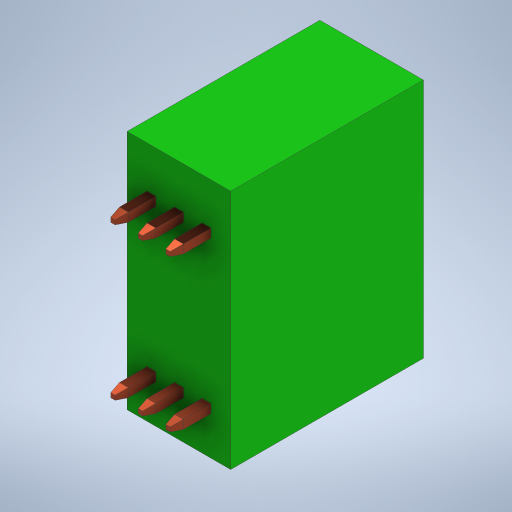
# Autodesk Inventor part: DB2EVH-2.5-2-3P-GN
Saved by Autodesk Inventor 2024 (Build 280153000, 153)
## iProperties
Created: 2023-05-23
Part Number: DB2EVH-2.5-2-3P-GN
Material: Generic
Document SubType Name: Modeling
Designer: torba
Density: 1 g/cm^3
Appearance: Default
Author: torba
Autodesk Inventor part; units mm, degrees
ref_plane "YZ Plane" through (0, 0, 0) normal (1, 0, 0) x (0, 1, 0)
ref_plane "XZ Plane" through (0, 0, 0) normal (0, 1, 0) x (-1, 0, 0)
ref_plane "XY Plane" through (0, 0, 0) normal (0, 0, 1) x (1, 0, 0)
sketch "Sketch1" plane through (0, 0, 0) normal (0, 0, 1) x (1, 0, 0)
  line L0 (0, 0) -> (9.4, 0)
  line L1 (9.4, 0) -> (9.4, -21.9)
  line L2 (9.4, -21.9) -> (0, -21.9)
  line L3 (0, -21.9) -> (0, 0)
  line L4 (1.8, -18.4) -> (2.6, -18.4)
  line L5 (2.6, -18.4) -> (2.6, -17.6)
  line L6 (2.6, -17.6) -> (1.8, -17.6)
  line L7 (1.8, -17.6) -> (1.8, -18.4)
  line L8 (1.8, -18.4) -> (2.6, -17.6) construction
  point P0 (2.2, -18)
  dimension "d0" = 9.4
  dimension "d1" = 21.9
  dimension "d2" = 0.8
  dimension "d3" = 0.8
  dimension "d5" = 3.9
  dimension "d6" = 2.2
  dimension "d14" = 0
  dimension "d15" = 0
  dimension "d22" = 7.2
  constraints: 18 end point, 4 parallel, 2 horizontal, 2 perpendicular, 1 midpoint
  measures "d0" distance between parallel lines of L1 L3
  measures "d1" distance between parallel lines of L2 L0
  measures "d2" distance of L4.end L5.end
  measures "d3" distance of L4.start L4.end
  measures "d5" distance from line of L2 point (2.2, -18)
  measures "d6" distance from line of L3 point (2.2, -18)
  measures "d14" distance from line of point (0, 0) L3
  measures "d15" distance from line of point (0, 0) L0
  measures "d22" distance from line of point (2.2, -18) L1
extrude "Extrusion1" add sketch "Sketch1" along normal blind 3.5 contours L7 L6 L5 L4
chamfer "Chamfer1" distance 0.2 distance2 1 4 edges at (2.6, -18, 3.5) (2.2, -18.4, 3.5) (1.8, -18, 3.5) (2.2, -17.6, 3.5) measured on face at (2.2, -17.9, 3.5) measured on face at (2.3, -18, 3.5) measured on face at (2.2, -18.1, 3.5) measured on face at (2.1, -18, 3.5)
extrude "Extrusion2" add sketch "Sketch1" against normal blind 17.5 separate body contours L0 L1 L2 L3 | L7 L6 L5 L4
pattern_linear "Rectangular Pattern1" count 2 spacing 13.8 along (0, 1, 0) count 3 spacing 2.5 along (1, 0, 0) of "Extrusion1", "Chamfer1" bodies 1
equation "\"d3\" = d2"
body "Solid1"
